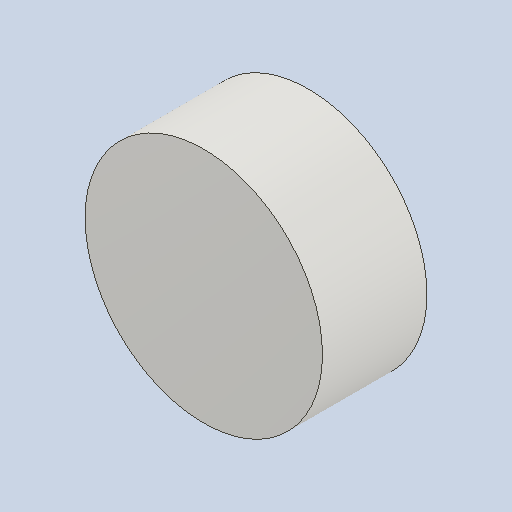
# Autodesk Inventor part: Koło pasowe zwykłe1
Saved by Autodesk Inventor 2023 (Build 270158000, 158)
## iProperties
CustomPartVersion: 1
Created: 2023-04-25
Part Number: Koło pasowe zwykłe1
Material: Steel
Document SubType Name: Modeling
Designer: krzys
Density: 7.85 g/cm^3
Appearance: Steel
Author: krzys
Autodesk Inventor part; units mm, degrees
ref_plane "YZ Plane" through (0, 0, 0) normal (1, 0, 0) x (0, 1, 0)
ref_plane "XZ Plane" through (0, 0, 0) normal (0, 1, 0) x (-1, 0, 0)
ref_plane "XY Plane" through (0, 0, 0) normal (0, 0, 1) x (1, 0, 0)
sketch "Szkic główny" plane through (0, 0, 0) normal (0, 0, 1) x (1, 0, 0)
  circle A0 centre (0, 0) radius 20
  dimension "d0" = 40
  constraints: 1 centre point, 1 coincident
  measures "d0" diameter of A0
extrude "Koło pasowe" add sketch "Szkic główny" along normal mid plane 17.6
equation "\"d0\" = da_D"
equation "\"d1\" = da_B"
equation "\"da_D\" = 40"
equation "\"da_B\" = 17.6"
body "Solid1"
